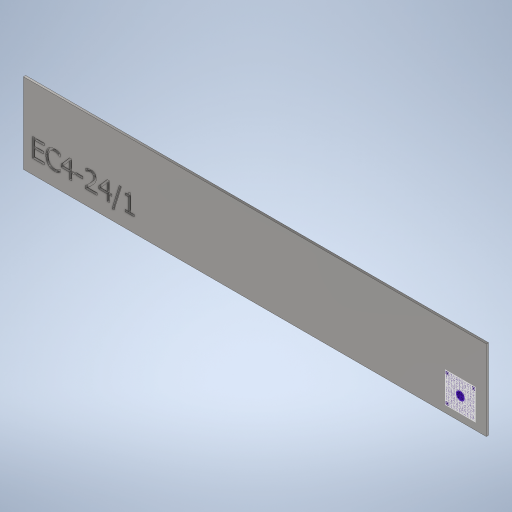
# Autodesk Inventor part: Fechamento
Saved by Autodesk Inventor 2024.2 (Build 282272000, 272)
## iProperties
Created: 2024-05-06
Part Number: Fechamento
Material: Steel, Alloy
Document SubType Name: Modeling
Designer: 082220005
Density: 7.73 g/cm^3
Appearance: Semi-Polished
Author: 082220005
Autodesk Inventor part; units mm, degrees
note: some values were not read from the file. Chosen so that the rebuilt part matches the saved one: direction of "Emboss2".
ref_plane "YZ Plane" through (0, 0, 0) normal (1, 0, 0) x (0, 1, 0)
ref_plane "XZ Plane" through (0, 0, 0) normal (0, 1, 0) x (-1, 0, 0)
sketch "Sketch1" plane through (0, 0, 0) normal (0, 0, 1) x (1, 0, 0)
  line L0 (0, 0) -> (75, 0)
  line L1 (75, 0) -> (75, 13)
  line L2 (75, 13) -> (0, 13)
  line L3 (0, 13) -> (0, 0)
  dimension "d0" = 75
  dimension "d1" = 13
  constraints: 8 end point, 3 perpendicular, 1 horizontal
  measures "d0" distance of L0.start L0.end
  measures "d1" distance of L0.end L1.end
extrude "Extrusion1" add sketch "Sketch1" along normal blind 0.3556
ref_plane "Work Plane2" through (0, 0, 17.3556) normal (0, 0, 1) x (1, 0, 0)
sketch "Sketch4" plane through (0, 0, 17.3556) normal (0, 0, 1) x (1, 0, 0)
  line L0 (67.9102, 5.6782) -> (72.9102, 5.6782) construction
  line L1 (72.9102, 5.6782) -> (72.9102, 0.6782) construction
  line L2 (72.9102, 0.6782) -> (67.9102, 0.6782) construction
  line L3 (67.9102, 0.6782) -> (67.9102, 5.6782) construction
  line L4 (1.1407, 5.4875) -> (34.0945, 5.4875) construction
  line L5 (34.0945, 5.4875) -> (34.0945, 1.5722) construction
  line L6 (34.0945, 1.5722) -> (1.1407, 1.5722) construction
  line L7 (1.1407, 1.5722) -> (1.1407, 5.4875) construction
  line L8 (1.4495, 2.3037) -> (1.4495, 5.3517)
  line L9 (1.4495, 5.3517) -> (3.3563, 5.3517)
  line L10 (3.3563, 5.3517) -> (3.3563, 4.9911)
  line L11 (3.3563, 4.9911) -> (1.8546, 4.9911)
  line L12 (1.8546, 4.9911) -> (1.8546, 4.1562)
  line L13 (1.8546, 4.1562) -> (3.2551, 4.1562)
  line L14 (3.2551, 4.1562) -> (3.2551, 3.7956)
  line L15 (3.2551, 3.7956) -> (1.8546, 3.7956)
  line L16 (1.8546, 3.7956) -> (1.8546, 2.6643)
  line L17 (1.8546, 2.6643) -> (3.3563, 2.6643)
  line L18 (3.3563, 2.6643) -> (3.3563, 2.3037)
  line L19 (3.3563, 2.3037) -> (1.4495, 2.3037)
  spline S0 degree 2 poles (4.9915, 2.2493) (4.6951, 2.2493) (4.1937, 2.4494) (4.0109, 2.6495) knots 0 0 0 1 2 2 2
  spline S1 degree 2 poles (4.0109, 2.6495) (3.8281, 2.8471) (3.6281, 3.4399) (3.6281, 3.8252) knots 0 0 0 1 2 2 2
  spline S2 degree 2 poles (3.6281, 3.8252) (3.6281, 4.2081) (3.8232, 4.7762) (4.0084, 4.9861) knots 0 0 0 1 2 2 2
  spline S3 degree 2 poles (4.0084, 4.9861) (4.1912, 5.1911) (4.6902, 5.406) (4.9989, 5.406) knots 0 0 0 1 2 2 2
  spline S4 degree 2 poles (4.9989, 5.406) (5.1521, 5.406) (5.4213, 5.3616) (5.5349, 5.327) knots 0 0 0 1 2 2 2
  spline S5 degree 2 poles (5.5349, 5.327) (5.6337, 5.2949) (5.8387, 5.2035) (5.94, 5.1491) knots 0 0 0 1 2 2 2
  line L20 (5.94, 5.1491) -> (5.94, 4.6601)
  line L21 (5.94, 4.6601) -> (5.9079, 4.6601)
  spline S6 degree 2 poles (5.9079, 4.6601) (5.8535, 4.7095) (5.6856, 4.8478) (5.5645, 4.9145) knots 0 0 0 1 2 2 2
  spline S7 degree 2 poles (5.5645, 4.9145) (5.4485, 4.9787) (5.1743, 5.0602) (4.9964, 5.0602) knots 0 0 0 1 2 2 2
  spline S8 degree 2 poles (4.9964, 5.0602) (4.8013, 5.0602) (4.453, 4.8997) (4.3221, 4.7465) knots 0 0 0 1 2 2 2
  spline S9 degree 2 poles (4.3221, 4.7465) (4.1937, 4.5909) (4.0504, 4.1191) (4.0504, 3.8252) knots 0 0 0 1 2 2 2
  spline S10 degree 2 poles (4.0504, 3.8252) (4.0504, 3.5115) (4.2011, 3.0595) (4.332, 2.9039) knots 0 0 0 1 2 2 2
  spline S11 degree 2 poles (4.332, 2.9039) (4.4604, 2.7532) (4.8038, 2.6001) (4.9964, 2.6001) knots 0 0 0 1 2 2 2
  spline S12 degree 2 poles (4.9964, 2.6001) (5.1718, 2.6001) (5.4707, 2.6865) (5.5868, 2.7508) knots 0 0 0 1 2 2 2
  spline S13 degree 2 poles (5.5868, 2.7508) (5.6979, 2.815) (5.8634, 2.9484) (5.9103, 2.9953) knots 0 0 0 1 2 2 2
  line L22 (5.9103, 2.9953) -> (5.94, 2.9953)
  line L23 (5.94, 2.9953) -> (5.94, 2.5112)
  spline S14 degree 2 poles (5.94, 2.5112) (5.8387, 2.4642) (5.6609, 2.3778) (5.5349, 2.3383) knots 0 0 0 1 2 2 2
  spline S15 degree 2 poles (5.5349, 2.3383) (5.4015, 2.2938) (5.1743, 2.2493) (4.9915, 2.2493) knots 0 0 0 1 2 2 2
  line L24 (8.1926, 3.351) -> (7.8295, 3.351)
  line L25 (7.8295, 3.351) -> (7.8295, 2.3037)
  line L26 (7.8295, 2.3037) -> (7.4368, 2.3037)
  line L27 (7.4368, 2.3037) -> (7.4368, 3.351)
  line L28 (7.4368, 3.351) -> (6.0907, 3.351)
  line L29 (6.0907, 3.351) -> (6.0907, 3.7808)
  line L30 (6.0907, 3.7808) -> (7.4541, 5.3517)
  line L31 (7.4541, 5.3517) -> (7.8295, 5.3517)
  line L32 (7.8295, 5.3517) -> (7.8295, 3.6795)
  line L33 (7.8295, 3.6795) -> (8.1926, 3.6795)
  line L34 (8.1926, 3.6795) -> (8.1926, 3.351)
  line L35 (7.4368, 3.6795) -> (7.4368, 4.87)
  line L36 (7.4368, 4.87) -> (6.4118, 3.6795)
  line L37 (6.4118, 3.6795) -> (7.4368, 3.6795)
  line L38 (9.6351, 3.4522) -> (8.4816, 3.4522)
  line L39 (8.4816, 3.4522) -> (8.4816, 3.8227)
  line L40 (8.4816, 3.8227) -> (9.6351, 3.8227)
  line L41 (9.6351, 3.8227) -> (9.6351, 3.4522)
  line L42 (11.9199, 2.3037) -> (10.0402, 2.3037)
  line L43 (10.0402, 2.3037) -> (10.0402, 2.7359)
  spline S16 degree 2 poles (10.0402, 2.7359) (10.2428, 2.9261) (10.6034, 3.2793) (10.7763, 3.4695) knots 0 0 0 1 2 2 2
  spline S17 degree 2 poles (10.7763, 3.4695) (11.1245, 3.8524) (11.379, 4.3118) (11.379, 4.5563) knots 0 0 0 1 2 2 2
  spline S18 degree 2 poles (11.379, 4.5563) (11.379, 4.6848) (11.2999, 4.8774) (11.2283, 4.9392) knots 0 0 0 1 2 2 2
  spline S19 degree 2 poles (11.2283, 4.9392) (11.1567, 5.0009) (10.9689, 5.0627) (10.8553, 5.0627) knots 0 0 0 1 2 2 2
  spline S20 degree 2 poles (10.8553, 5.0627) (10.7466, 5.0627) (10.5243, 5.0083) (10.4231, 4.9664) knots 0 0 0 1 2 2 2
  spline S21 degree 2 poles (10.4231, 4.9664) (10.3366, 4.9318) (10.1761, 4.833) (10.1267, 4.7984) knots 0 0 0 1 2 2 2
  line L44 (10.1267, 4.7984) -> (10.1044, 4.7984)
  line L45 (10.1044, 4.7984) -> (10.1044, 5.2331)
  spline S22 degree 2 poles (10.1044, 5.2331) (10.2304, 5.2949) (10.6824, 5.4159) (10.885, 5.4159) knots 0 0 0 1 2 2 2
  spline S23 degree 2 poles (10.885, 5.4159) (11.3123, 5.4159) (11.7939, 4.9639) (11.7939, 4.5786) knots 0 0 0 1 2 2 2
  spline S24 degree 2 poles (11.7939, 4.5786) (11.7939, 4.3983) (11.7099, 4.0969) (11.6358, 3.9685) knots 0 0 0 1 2 2 2
  spline S25 degree 2 poles (11.6358, 3.9685) (11.5617, 3.8351) (11.3469, 3.5733) (11.2283, 3.4473) knots 0 0 0 1 2 2 2
  spline S26 degree 2 poles (11.2283, 3.4473) (11.0356, 3.2373) (10.5639, 2.7878) (10.4231, 2.6569) knots 0 0 0 1 2 2 2
  line L46 (10.4231, 2.6569) -> (11.9199, 2.6569)
  line L47 (11.9199, 2.6569) -> (11.9199, 2.3037)
  line L48 (14.2886, 3.351) -> (13.9255, 3.351)
  line L49 (13.9255, 3.351) -> (13.9255, 2.3037)
  line L50 (13.9255, 2.3037) -> (13.5328, 2.3037)
  line L51 (13.5328, 2.3037) -> (13.5328, 3.351)
  line L52 (13.5328, 3.351) -> (12.1867, 3.351)
  line L53 (12.1867, 3.351) -> (12.1867, 3.7808)
  line L54 (12.1867, 3.7808) -> (13.5501, 5.3517)
  line L55 (13.5501, 5.3517) -> (13.9255, 5.3517)
  line L56 (13.9255, 5.3517) -> (13.9255, 3.6795)
  line L57 (13.9255, 3.6795) -> (14.2886, 3.6795)
  line L58 (14.2886, 3.6795) -> (14.2886, 3.351)
  line L59 (13.5328, 3.6795) -> (13.5328, 4.87)
  line L60 (13.5328, 4.87) -> (12.5078, 3.6795)
  line L61 (12.5078, 3.6795) -> (13.5328, 3.6795)
  line L62 (15.8818, 5.4875) -> (14.6888, 1.6417)
  line L63 (14.6888, 1.6417) -> (14.343, 1.6417)
  line L64 (14.343, 1.6417) -> (15.5311, 5.4875)
  line L65 (15.5311, 5.4875) -> (15.8818, 5.4875)
  line L66 (17.9443, 2.3037) -> (16.4573, 2.3037)
  line L67 (16.4573, 2.3037) -> (16.4573, 2.6149)
  line L68 (16.4573, 2.6149) -> (17.0106, 2.6149)
  line L69 (17.0106, 2.6149) -> (17.0106, 4.6576)
  line L70 (17.0106, 4.6576) -> (16.4573, 4.6576)
  line L71 (16.4573, 4.6576) -> (16.4573, 4.9367)
  spline S27 degree 2 poles (16.4573, 4.9367) (16.771, 4.9367) (17.0674, 5.1146) (17.0872, 5.3616) knots 0 0 0 1 2 2 2
  line L72 (17.0872, 5.3616) -> (17.4033, 5.3616)
  line L73 (17.4033, 5.3616) -> (17.4033, 2.6149)
  line L74 (17.4033, 2.6149) -> (17.9443, 2.6149)
  line L75 (17.9443, 2.6149) -> (17.9443, 2.3037)
  point P0 (0, 0)
  dimension "d34" = 5
  constraints: 4 other
  measures "d34" distance of L0.start L0.end
emboss "Emboss2" sketch "Sketch4" operation cut depth 0.3 direction (0, 0, -1)
sketch "Sketch5" plane through (0, 0, 17.3556) normal (0, 0, 1) x (1, 0, 0)
  line L0 (68.2954, 6.0931) -> (73.2954, 6.0931) construction
  line L1 (73.2954, 6.0931) -> (73.2954, 1.0931) construction
  line L2 (73.2954, 1.0931) -> (68.2954, 1.0931) construction
  line L3 (68.2954, 1.0931) -> (68.2954, 6.0931) construction
  point P0 (0, 0)
  dimension "d50" = 5
  constraints: 2 other
  measures "d50" distance of L0.start L0.end
decal "Decal2"
body "Solid1"
